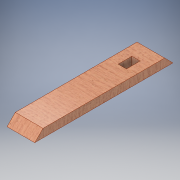
# Autodesk Inventor part: Front
Saved by Autodesk Inventor 2019.3 (Build 233278000, 278)
## iProperties
Created: 2019-01-12
Part Number: Front
Material: Holz (Eiche)
Document SubType Name: Modeling
Designer: Jonas
Density: 0.76 g/cm^3
Appearance: Weißeiche - natur - mittlerer Glanz
Author: Jonas
Autodesk Inventor part; units mm, degrees
ref_plane "YZ Plane" through (0, 0, 0) normal (1, 0, 0) x (0, 1, 0)
ref_plane "XZ Plane" through (0, 0, 0) normal (0, 1, 0) x (-1, 0, 0)
ref_plane "XY Plane" through (0, 0, 0) normal (0, 0, 1) x (1, 0, 0)
sketch "Skizze1" plane through (0, 0, 0) normal (0, 1, 0) x (-1, 0, 0)
  line L0 (35.9259, 133.0751) -> (-24.0741, 133.0751)
  line L1 (-24.0741, 133.0751) -> (-24.0741, -166.9249)
  line L2 (-24.0741, -166.9249) -> (35.9259, -166.9249)
  line L3 (35.9259, -166.9249) -> (35.9259, 133.0751)
  point P0 (0, 0)
  dimension "d0" = 60
  dimension "d1" = 300
  constraints: 8 end point, 2 parallel, 1 horizontal, 1 perpendicular
  measures "d0" distance of L0.start L0.end
  measures "d1" distance of L2.end L0.start
extrude "Extrusion1" add sketch "Skizze1" along normal blind 18
chamfer "Fase1" distance 18 angle 45 1 edges at (-5.9259, 18, 133.0751)
chamfer "Fase2" distance 18 angle 45 1 edges at (-5.9259, 18, -166.9249)
sketch "Skizze4" plane through (0, 0, 0) normal (0, -1, 0) x (1, 0, 0)
  line L0 (-14.9259, -116.9249) -> (3.0741, -116.9249)
  line L1 (3.0741, -116.9249) -> (3.0741, -86.9249)
  line L2 (3.0741, -86.9249) -> (-14.9259, -86.9249)
  line L3 (-14.9259, -86.9249) -> (-14.9259, -116.9249)
  line L4 (-14.9259, -116.9249) -> (3.0741, -86.9249) construction
  line L5 (3.0741, -116.9249) -> (-14.9259, -86.9249) construction
  line L6 (-35.9259, -166.9249) -> (-35.9259, 133.0751) projected
  line L7 (24.0741, -166.9249) -> (-35.9259, -166.9249) projected
  point P0 (-5.9259, -101.9249)
  dimension "d28" = 30
  dimension "d29" = 30
  dimension "d30" = 18
  dimension "d31" = 50
  constraints: 12 end point, 2 midpoint, 2 parallel, 1 horizontal, 1 perpendicular
  measures "d28" distance from line of L6 point (-5.926, -101.925)
  measures "d29" distance of L2.end L0.start
  measures "d30" distance of L1.end L2.end
  measures "d31" distance between parallel lines of L7 L0
extrude "Extrusion2" cut sketch "Skizze4" against normal blind 18
sketch "Skizze2" plane through (0, 18, 0) normal (0, 1, 0) x (1, 0, 0)
  point P0 (38.0741, -40.5751)
sketch "Skizze3" plane through (0, 18, 0) normal (0, 1, 0) x (1, 0, 0)
  point P0 (38.0741, 74.4249)
sketch "Skizze5" plane through (0, 0, 0) normal (0, -1, 0) x (1, 0, 0)
  point P0 (-5.9259, -122.9249)
hole "Bohrung5" at (-5.9259, 0, -122.9249) direction (0, 1, 0) diameter 2.459 depth 8 tip angle 120 thread size "M3x0.5" class "6H" standard "ISO Metric profile"
sketch "Skizze6" plane through (0, 0, 0) normal (0, -1, 0) x (1, 0, 0)
  point P0 (-5.9259, -81.7341)
hole "Bohrung7" at (-5.9259, 0, -81.7341) direction (0, 1, 0) diameter 2.459 depth 8 tip angle 120 thread size "M3x0.5" class "6H" standard "ISO Metric profile"
